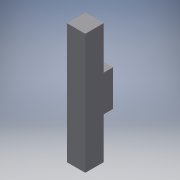
# Autodesk Inventor part: PiezaPuerta-1
Saved by Autodesk Inventor 2017 (Build 210142000, 142)
## iProperties
Created: 2021-02-12
Part Number: PiezaPuerta-1
Material: Generic
Document SubType Name: Modeling
Designer: USUARIO
Density: 1 g/cm^3
Appearance: Default
Author: USUARIO
Autodesk Inventor part; units mm, degrees
ref_plane "YZ Plane" through (0, 0, 0) normal (1, 0, 0) x (0, 1, 0)
ref_plane "XZ Plane" through (0, 0, 0) normal (0, 1, 0) x (-1, 0, 0)
ref_plane "XY Plane" through (0, 0, 0) normal (0, 0, 1) x (1, 0, 0)
sketch "Sketch1" plane through (0, 0, 0) normal (0, 1, 0) x (-1, 0, 0)
  line L0 (0, 0) -> (50.8, 0)
  line L1 (50.8, 0) -> (50.8, -334)
  line L2 (50.8, -334) -> (0, -334)
  line L3 (0, -334) -> (0, 0)
  dimension "d0" = 50.8
  dimension "d1" = 334
  constraints: 8 end point, 2 parallel, 1 horizontal, 1 perpendicular
  measures "d0" distance of L1.end L2.end
  measures "d1" distance of L0.end L1.end
extrude "Extrusion1" add sketch "Sketch1" along normal blind 77
sketch "Sketch3" plane through (0, 0, 0) normal (1, 0, 0) x (0, 0, -1)
  line L0 (0, 77) -> (121, 77)
  line L1 (121, 77) -> (121, 51.2)
  line L2 (121, 51.2) -> (0, 51.2)
  line L3 (0, 51.2) -> (0, 77)
  line L4 (0, 77) -> (334, 77) projected
  line L5 (334, 77) -> (217, 77)
  line L6 (217, 77) -> (217, 51.2)
  line L7 (217, 51.2) -> (334, 51.2)
  line L8 (334, 51.2) -> (334, 77)
  point P0 (0, 0)
  dimension "d9" = 25.8
  dimension "d10" = 117
  dimension "d11" = 25.8
  dimension "d14" = 96
  constraints: 16 end point, 4 parallel, 2 horizontal, 2 perpendicular
  measures "d9" distance of L0.end L1.end
  measures "d10" distance of L7.end L6.end
  measures "d11" distance of L6.end L5.end
  measures "d14" distance between parallel lines of L1 L6
extrude "Extrusion2" cut sketch "Sketch3" against normal blind 50.8
body "Solid1"
